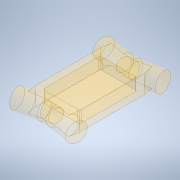
# Autodesk Inventor part: soft_body_v2_simplified
Saved by Autodesk Inventor 2020.2 (Build 242310000, 310)
## iProperties
Created: 2020-07-17
Part Number: soft_body_v2_simplified
Material: Generic
Document SubType Name: Modeling
Designer: boxi
Density: 1 g/cm^3
Appearance: Default
Mass: 1916.47 g
Surface Area: 2811.02 cm^2
Volume: 1916.47 cm^3
Author: boxi
Autodesk Inventor part; units mm, degrees
ref_plane "YZ Plane" through (0, 0, 0) normal (1, 0, 0) x (0, 1, 0)
ref_plane "XY Plane" through (0, 0, 0) normal (0, 0, 1) x (1, 0, 0)
sketch "Sketch1" plane through (0, 0, 0) normal (0, 1, 0) x (-1, 0, 0)
  line L0 (142.9941, 155.2137) -> (0, 130) construction
  line L1 (0, -43.5293) -> (0, 245.4256) projected
  line L2 (256.6466, 0) -> (-100.8661, 0) projected
  line L3 (90.4845, 132.2466) -> (91.6133, 125.8454)
  line L4 (91.6133, 125.8454) -> (98.0145, 126.9741)
  line L5 (98.0145, 126.9741) -> (98.1882, 125.9893)
  line L6 (98.1882, 125.9893) -> (105.0818, 127.2048)
  line L7 (105.0818, 127.2048) -> (106.9919, 116.3719)
  line L8 (106.9919, 116.3719) -> (23.2833, 101.6118)
  line L9 (90.4845, 132.2466) -> (87.5301, 131.7257)
  line L10 (85.5605, 131.3784) -> (86.8629, 123.9923)
  line L11 (86.8629, 123.9923) -> (50.425, 117.5673)
  line L12 (50.425, 117.5673) -> (48.4669, 114.1758)
  line L13 (48.4669, 114.1758) -> (21.8941, 109.4903)
  line L14 (87.5301, 131.7257) -> (89.1103, 122.7639)
  line L15 (89.1103, 122.7639) -> (51.7447, 116.1753)
  line L16 (51.7447, 116.1753) -> (48.7447, 112.6001)
  line L17 (48.7447, 112.6001) -> (22.1719, 107.9146)
  line L18 (21.8941, 109.4903) -> (22.1719, 107.9146)
  line L19 (22.1719, 107.9146) -> (23.2833, 101.6118)
  line L20 (69.4433, 142.2447) -> (75, 110.7309)
  line L21 (75, 107.3146) -> (75, 0)
  line L22 (17.7265, 133.1257) -> (85.1859, 145.0206)
  line L23 (17.7265, 133.1257) -> (21.8941, 109.4903)
  line L24 (87.5301, 131.7257) -> (85.5605, 131.3784)
  line L25 (85.1859, 145.0206) -> (87.5301, 131.7257)
  line L26 (23.2833, 101.6118) -> (0, 101.6118) construction
  line L27 (75, 110.7309) -> (75, 107.3146)
  line L28 (17.7265, 133.1257) -> (0, 130)
  line L29 (67, 0) -> (67, 92.5146)
  line L30 (86.8629, 123.9923) -> (49.4402, 117.3937) construction
  line L31 (49.4402, 117.3937) -> (45.7936, 138.0746) construction
  line L32 (49.4402, 117.3937) -> (39.5921, 115.6572) construction
  line L33 (39.5921, 115.6572) -> (35.9455, 136.3382) construction
  line L34 (39.5921, 115.6572) -> (16.9415, 111.6633) construction
  line L35 (16.9415, 111.6633) -> (13.2949, 132.3443) construction
  line L36 (46.1903, 116.8206) -> (42.5437, 137.5016) construction
  line L37 (42.1526, 116.1087) -> (38.506, 136.7896) construction
  line L38 (0, 55) -> (28, 55)
  line L39 (40, 43) -> (40, 0)
  arc A0 (40, 43) -> (28, 55) centre (28, 43) ccw
  line L40 (75, 107.3146) -> (0, 107.3146)
  line L41 (21.8941, 109.4903) -> (0, 109.4903)
  line L42 (0, 102.5146) -> (57, 102.5146)
  line L43 (17.7265, 133.1257) -> (0, 133.1257)
  line L44 (0, 55) -> (-28, 55)
  line L45 (-40, 43) -> (-40, 0)
  arc A1 (-28, 55) -> (-40, 43) centre (-28, 43) ccw
  line L46 (17.7265, 133.1257) -> (13.559, 156.7611) construction
  line L47 (13.559, 156.7611) -> (46.6849, 162.602) construction
  line L48 (13.559, 156.7611) -> (12.1698, 164.6395) construction
  line L49 (12.1698, 164.6395) -> (95.8785, 179.3996) construction
  line L50 (21.7552, 110.2781) -> (24.5126, 110.7643)
  line L51 (24.5126, 110.7643) -> (25.5905, 110.1421)
  arc A2 (67, 92.5146) -> (57, 102.5146) centre (57, 92.5146) ccw
  line L52 (75, 115.3146) -> (0, 115.3146)
  circle A3 centre (42.5, 0) radius 1.25
  line L53 (45, 0) -> (45, 43)
  arc A4 (45, 43) -> (28, 60) centre (28, 43) ccw
  line L54 (28, 60) -> (0, 60)
  line L55 (0, 60) -> (-28, 60)
  arc A5 (-28, 60) -> (-45, 43) centre (-28, 43) ccw
  line L56 (-45, 43) -> (-45, 0)
  circle A6 centre (42.5, 0) radius 2.25
  line L57 (45, 0) -> (40, 0) construction
  circle A7 centre (0, 57.5) radius 1.25
  circle A8 centre (0, 57.5) radius 2.25
  line L58 (105.0818, 127.2048) -> (101.4352, 147.8858)
  line L59 (85.1859, 145.0206) -> (101.4352, 147.8858)
  line L60 (142.9941, 155.2137) -> (173.3904, -17.1725) construction
  line L61 (12.1698, 164.6395) -> (0, 164.6395) construction
  point P0 (73.3677, 119.9881)
  point P1 (73.0899, 121.5638)
  point P2 (0, 0)
  point P3 (55.6253, 107.3146)
  point P4 (22.2777, 107.3146)
  point P5 (26.6933, 125.6494)
  point P6 (15.6506, 125.6494)
  point P7 (74.1918, 115.3146)
  point P8 (103.6018, 148.2678)
  point P9 (149.94, 115.8214)
  point P10 (74.9102, 105.4662)
  point P11 (0, 59.75)
  point P12 (0, 55.25)
  point P13 (40.25, 0)
  point P14 (44.75, 0)
  dimension "d340" = 10
  dimension "d353" = 1
  dimension "d440" = 10
  dimension "d443" = 10
  dimension "d446" = 4.942
  dimension "d0" = 10
  dimension "d1" = 1
  dimension "d3" = 50
  dimension "d4" = 3
  dimension "d5" = 37
  dimension "d6" = 2
  dimension "d7" = 1.6
  dimension "d9" = 1.6
  dimension "d10" = 42
  dimension "d11" = 6.5
  dimension "d12" = 7
  dimension "d13" = 27
  dimension "d14" = 3
  dimension "d15" = 42
  dimension "d16" = 6.4
  dimension "d17" = 260
  dimension "d24" = 64
  dimension "d27" = 35.4531
  dimension "d63" = 8
  dimension "d67" = 38
  dimension "d68" = 10
  dimension "d69" = 23
  dimension "d77" = 4.1
  dimension "d78" = 3.3
  dimension "d122" = 12
  dimension "d128" = 110
  dimension "d129" = 80
  dimension "d144" = 48
  dimension "d161" = 4.8
  dimension "d190" = 214.6292
  dimension "d193" = 9.4
  dimension "d224" = 45.2
  dimension "d225" = 29.5
  dimension "d226" = 1.6
  dimension "d227" = 40
  dimension "d324" = 40
  dimension "d325" = 0.8
  dimension "d326" = 2.8
  dimension "d456" = 10
  dimension "d468" = 11
  dimension "d469" = 24.3396
  dimension "d513" = 32.4855
  dimension "d514" = 8
  dimension "d520" = 230.6292
  dimension "d538" = 150
  dimension "d539" = 4.5
  dimension "d543" = 0.6
  dimension "d545" = 2.5
  dimension "d546" = 5
  dimension "d548" = 4.5
  dimension "d676" = 2.5
  dimension "d717" = 85
  dimension "d718" = 103
  dimension "d721" = 134
  dimension "d724" = 18
  dimension "d725" = 358.7992
  dimension "d726" = 175.0455
  dimension "d727" = 2.2
  dimension "d728" = 40
  dimension "d729" = 40
  dimension "d730" = 135.0455
  dimension "d731" = 346.7808
  dimension "d732" = 285.9882
  dimension "d733" = 90
  constraints: 120 end point, 14 point on line, 10 point on circle, 9 centre point, 8 horizontal, 6 perpendicular, 4 coincident, 4 horizontal alignment, 4 tangent, 3 equal radius, 3 vertical, 2 collinear, 2 parallel, 1 midpoint, 60 other
  measures "d1" distance between parallel lines of L6 L4
  measures "d3" angle of L12 L11
  measures "d4" distance from line of L13 L11.end
  measures "d5" distance of L10.end L11.end
  measures "d6" distance between parallel lines of L14 L10
  measures "d7" distance between parallel lines of L15 L11
  measures "d9" distance between parallel lines of L17 L13
  measures "d11" distance of L3.end L4.end
  measures "d12" distance of L5.end L6.end
  measures "d14" distance between parallel lines of L3 L14
  measures "d16" distance between parallel lines of L8 L17
  measures "d17" diameter of L28.end L2
  measures "d63" distance between parallel lines of L29 L21
  measures "d67" distance of L10.end L30.end
  measures "d68" distance between parallel lines of L31 L33
  measures "d69" distance of L32.end L34.end
  measures "d77" distance between parallel lines of L36 L37
  measures "d78" distance between parallel lines of L31 L36
  measures "d122" radius of A0
  measures "d128" diameter of L38 L2
  measures "d161" distance between parallel lines of L42 L40
  measures "d190" diameter of L21.start L2
  measures "d193" distance between parallel lines of L8 L15
  measures "d225" distance from line of L23 L11.end
  measures "d226" distance of L16.end L12.end
  measures "d227" angle of L16 L15
  measures "d324" angle of L13 L51
  measures "d325" distance between parallel lines of L13 L50
  measures "d326" distance of L50.start L50.end
  measures "d456" radius of A2
  measures "d468" distance between parallel lines of L8 L6
  measures "d513" distance between parallel lines of L7 L20
  measures "d514" distance from line of L40 L52.start
  measures "d520" diameter of L52.start L2
  measures "d539" distance between parallel lines of L35 L23
  measures "d543" distance from line of L40 L17.end
  measures "d545" diameter of A3
  measures "d546" distance between parallel lines of L39 L53
  measures "d548" diameter of A6
  measures "d676" distance from line of L44 A7.centre
  measures "d717" distance of L58.end L22.start
  measures "d718" distance of L58.end L28.end
  measures "d724" distance of L22.start L28.end
  measures "d725" diameter of L49.end L2
  measures "d727" distance from line of L58 point (103.602, 148.268)
  measures "d728" distance from line of point (103.602, 148.268) L60
  measures "d730" distance of L60.end point (149.94, 115.821)
sketch "Sketch24" plane through (0, 0, 0) normal (0, 1, 0) x (-1, 0, 0)
  line L0 (482.6663, 0) -> (-138.5361, 0) projected
  line L1 (0, -519.9214) -> (0, 362.0665) projected
  line L2 (75, 0) -> (144.4593, -393.9231)
  line L3 (0, 164.6395) -> (393.9231, 234.0988)
  point P0 (0, 0)
  dimension "d736" = 80
  dimension "d737" = 80
  dimension "d740" = 400
  dimension "d741" = 400
  constraints: 4 end point
  measures "d736" angle of L0 L2
  measures "d737" angle of L1 L3
  measures "d740" distance of L2.start L2.end
  measures "d741" distance of L3.start L3.end
sketch "Sketch_3_division_plane" plane through (0, 0, 0) normal (0, 1, 0) x (-1, 0, 0)
  line L0 (17.7265, 133.1257) -> (0, 133.1257) projected
  line L1 (17.7265, 133.1257) -> (172.7798, 160.4657)
  point P0 (0, 0)
  dimension "d207" = 10
  constraints: 2 end point
  measures "d207" angle of L1 L0
ref_plane "Work Plane5" through (-142.9941, 0, 155.2137) normal (0.1736482, 0, 0.9848078) x (0.9848078, 0, -0.1736482)
ref_plane "Work Plane4" through (-17.7265, 0, 133.1257) normal (-0.9848078, 0, 0.1736482) x (0, -1, 0)
ref_plane "Work Plane7" through (-17.7265, 0, 133.1257) normal (0, 0, 1) x (1, 0, 0)
sketch "Sketch2" plane through (-17.7265, 0, 133.1257) normal (-0.9848078, 0, 0.1736482) x (0, -1, 0)
  circle A0 centre (0, 0) radius 32
  circle A1 centre (0, 0) radius 24
  line L0 (-25.6, -10.6039) -> (-25.6, 10.6039)
  line L1 (-25.6, 10.6039) -> (-10.6039, 25.6)
  line L2 (-10.6039, 25.6) -> (10.6039, 25.6)
  line L3 (10.6039, 25.6) -> (25.6, 10.6039)
  line L4 (25.6, 10.6039) -> (25.6, -10.6039)
  line L5 (25.6, -10.6039) -> (10.6039, -25.6)
  line L6 (10.6039, -25.6) -> (-10.6039, -25.6)
  line L7 (-10.6039, -25.6) -> (-25.6, -10.6039)
  point P0 (0, -128.025)
  point P1 (0, 0)
  point P2 (0, 0)
  point P3 (0, 0)
  point P4 (0, -24)
  point P5 (0, -24)
  point P6 (0, -24)
  point P7 (0, -25.6)
  point P8 (0, -25.6)
  point P9 (0, -25.6)
  point P10 (0, -32)
  point P11 (0, -32)
  point P12 (0, -32)
  constraints: 16 end point, 3 coincident, 2 vertical alignment, 1 midpoint, 1 vertical, 21 other
sketch "Sketch3" plane through (0, 0, 0) normal (1, 0, 0) x (0, 1, 0)
  circle A0 centre (0, 133.1257) radius 22.6
  circle A1 centre (0, 133.1257) radius 32
  circle A2 centre (0, 133.1257) radius 28
  dimension "d162" = 64
  dimension "d163" = 45.2
  dimension "d460" = 4
  constraints: 3 centre point, 3 coincident
  measures "d162" diameter of A1
  measures "d163" diameter of A0
  measures "d460" radial gap between concentric circles of A1 A2
sketch "Sketch4" plane through (-142.9941, 0, 155.2137) normal (0.1736482, 0, 0.9848078) x (0.9848078, 0, -0.1736482)
  line L0 (102, 0) -> (106.1, 0) construction
  line L1 (107.55, -16) -> (100.55, -16)
  line L2 (100.55, -16) -> (100.55, 16)
  line L3 (100.55, 16) -> (107.55, 16)
  line L4 (107.55, 16) -> (107.55, -16)
  line L5 (107.55, -16) -> (100.55, 16) construction
  line L6 (100.55, -16) -> (107.55, 16) construction
  circle A0 centre (92.642, 27.3) radius 1.55
  line L7 (0, 0) -> (145.2, 0) construction
  circle A1 centre (92.642, 27.3) radius 1.25
  circle A2 centre (92.642, 27.3) radius 2.5
  line L8 (106.55, 16) -> (106.55, -16)
  line L9 (101.55, 16) -> (101.55, -16)
  line L10 (106.55, 16) -> (101.55, 16)
  line L11 (106.55, 15.3372) -> (106.55, -15.3372)
  line L12 (78.7206, 1.5) -> (77.6794, 1.5)
  line L13 (74.7, 4) -> (74.7, 5)
  line L14 (77.6794, 7.5) -> (78.7206, 7.5)
  line L15 (81.7, 5) -> (81.7, 4)
  line L16 (78.7206, 7.5) -> (81.7, 5)
  line L17 (81.7, 4) -> (78.7206, 1.5)
  line L18 (77.6794, 7.5) -> (74.7, 5)
  line L19 (77.6794, 1.5) -> (74.7, 4)
  line L20 (67.6794, 7.5) -> (64.7, 5)
  line L21 (67.6794, 7.5) -> (68.7206, 7.5)
  line L22 (68.7206, 7.5) -> (71.7, 5)
  line L23 (64.7, 4) -> (64.7, 5)
  line L24 (71.7, 5) -> (71.7, 4)
  line L25 (67.6794, 1.5) -> (64.7, 4)
  line L26 (71.7, 4) -> (68.7206, 1.5)
  line L27 (68.7206, 1.5) -> (67.6794, 1.5)
  line L28 (107.442, -7.8495) -> (106.442, -7.8495)
  line L29 (103.642, -5.5) -> (103.642, -4.5)
  line L30 (106.442, -2.1505) -> (107.442, -2.1505)
  line L31 (110.242, -4.5) -> (110.242, -5.5)
  line L32 (110.242, -5.5) -> (107.442, -7.8495)
  line L33 (110.242, -4.5) -> (107.442, -2.1505)
  line L34 (106.442, -7.8495) -> (103.642, -5.5)
  line L35 (106.442, -2.1505) -> (103.642, -4.5)
  line L36 (110.242, -5) -> (103.642, -5) construction
  line L37 (106.942, -7.8495) -> (106.942, -2.1505) construction
  line L38 (106.442, 2.1505) -> (103.642, 4.5)
  line L39 (103.642, 4.5) -> (103.642, 5.5)
  line L40 (106.442, 7.8495) -> (103.642, 5.5)
  line L41 (106.942, 2.1505) -> (106.942, 7.8495) construction
  line L42 (107.442, 2.1505) -> (106.442, 2.1505)
  line L43 (106.442, 7.8495) -> (107.442, 7.8495)
  line L44 (110.242, 5) -> (103.642, 5) construction
  line L45 (110.242, 4.5) -> (107.442, 2.1505)
  line L46 (110.242, 5.5) -> (110.242, 4.5)
  line L47 (110.242, 5.5) -> (107.442, 7.8495)
  line L48 (118.442, -7.8495) -> (115.642, -5.5)
  line L49 (115.642, -5.5) -> (115.642, -4.5)
  line L50 (118.442, -2.1505) -> (115.642, -4.5)
  line L51 (118.942, -7.8495) -> (118.942, -2.1505) construction
  line L52 (119.442, -7.8495) -> (118.442, -7.8495)
  line L53 (118.442, -2.1505) -> (119.442, -2.1505)
  line L54 (122.242, -5) -> (115.642, -5) construction
  line L55 (122.242, -5.5) -> (119.442, -7.8495)
  line L56 (122.242, -4.5) -> (122.242, -5.5)
  line L57 (122.242, -4.5) -> (119.442, -2.1505)
  line L58 (118.442, 2.1505) -> (115.642, 4.5)
  line L59 (115.642, 4.5) -> (115.642, 5.5)
  line L60 (118.442, 7.8495) -> (115.642, 5.5)
  line L61 (118.942, 2.1505) -> (118.942, 7.8495) construction
  line L62 (119.442, 2.1505) -> (118.442, 2.1505)
  line L63 (118.442, 7.8495) -> (119.442, 7.8495)
  line L64 (122.242, 5) -> (115.642, 5) construction
  line L65 (122.242, 4.5) -> (119.442, 2.1505)
  line L66 (122.242, 5.5) -> (122.242, 4.5)
  line L67 (122.242, 5.5) -> (119.442, 7.8495)
  line L68 (107.55, 13) -> (100.55, 13)
  line L69 (107.55, -13) -> (100.55, -13)
  line L70 (81.7, 4.5) -> (74.7, 4.5) construction
  line L71 (78.7206, -1.5) -> (77.6794, -1.5)
  line L72 (74.7, -4) -> (74.7, -5)
  line L73 (77.6794, -7.5) -> (78.7206, -7.5)
  line L74 (81.7, -5) -> (81.7, -4)
  line L75 (78.7206, -7.5) -> (81.7, -5)
  line L76 (81.7, -4) -> (78.7206, -1.5)
  line L77 (77.6794, -7.5) -> (74.7, -5)
  line L78 (77.6794, -1.5) -> (74.7, -4)
  line L79 (67.6794, -7.5) -> (64.7, -5)
  line L80 (67.6794, -7.5) -> (68.7206, -7.5)
  line L81 (68.7206, -7.5) -> (71.7, -5)
  line L82 (64.7, -4) -> (64.7, -5)
  line L83 (71.7, -5) -> (71.7, -4)
  line L84 (67.6794, -1.5) -> (64.7, -4)
  line L85 (71.7, -4) -> (68.7206, -1.5)
  line L86 (68.7206, -1.5) -> (67.6794, -1.5)
  line L87 (81.7, -4.5) -> (74.7, -4.5) construction
  line L88 (91.7, -4) -> (88.7206, -1.5)
  line L89 (88.7206, 7.5) -> (91.7, 5)
  line L90 (88.7206, -1.5) -> (87.6794, -1.5)
  line L91 (87.6794, -1.5) -> (84.7, -4)
  line L92 (84.7, -4) -> (84.7, -5)
  line L93 (91.7, -4.5) -> (84.7, -4.5) construction
  line L94 (87.6794, -7.5) -> (84.7, -5)
  line L95 (91.7, -5) -> (91.7, -4)
  line L96 (87.6794, -7.5) -> (88.7206, -7.5)
  line L97 (88.7206, -7.5) -> (91.7, -5)
  line L98 (88.7206, 1.5) -> (87.6794, 1.5)
  line L99 (84.7, 4) -> (84.7, 5)
  line L100 (87.6794, 7.5) -> (88.7206, 7.5)
  line L101 (91.7, 5) -> (91.7, 4)
  line L102 (91.7, 4) -> (88.7206, 1.5)
  line L103 (91.7, 4.5) -> (84.7, 4.5) construction
  line L104 (87.6794, 1.5) -> (84.7, 4)
  line L105 (87.6794, 7.5) -> (84.7, 5)
  line L106 (107.55, -16) -> (111.55, -16)
  line L107 (111.55, -16) -> (111.55, 16)
  line L108 (111.55, 16) -> (107.55, 16)
  line L109 (111.55, -5) -> (121.55, -5)
  line L110 (121.55, -5) -> (121.55, 5)
  line L111 (121.55, 5) -> (111.55, 5)
  line L112 (92.642, 27.3) -> (52.642, 27.3)
  circle A3 centre (52.642, 27.3) radius 1.25
  circle A4 centre (52.642, 27.3) radius 1.55
  circle A5 centre (52.642, 27.3) radius 2.5
  point P0 (167.7743, 0)
  point P1 (102, 0)
  point P2 (106.1, 0)
  point P3 (104.05, 0)
  point P4 (96.642, 0)
  point P5 (104.05, 16)
  point P6 (60.7, 0)
  point P7 (81.7, 1.5)
  point P8 (74.7, 7.5)
  point P9 (74.7, 1.5)
  point P10 (81.7, 7.5)
  point P11 (71.7, 7.5)
  point P12 (64.7, 7.5)
  point P13 (64.7, 1.5)
  point P14 (71.7, 1.5)
  point P15 (127.2, 0)
  point P16 (127.2, 0)
  point P17 (127.2, 0)
  point P18 (110.242, -7.8495)
  point P19 (103.642, -2.1505)
  point P20 (103.642, -7.8495)
  point P21 (110.242, -2.1505)
  point P22 (103.642, 2.1505)
  point P23 (103.642, 7.8495)
  point P24 (110.242, 2.1505)
  point P25 (110.242, 7.8495)
  point P26 (115.642, -7.8495)
  point P27 (115.642, -2.1505)
  point P28 (122.242, -7.8495)
  point P29 (122.242, -2.1505)
  point P30 (115.642, 2.1505)
  point P31 (115.642, 7.8495)
  point P32 (122.242, 2.1505)
  point P33 (122.242, 7.8495)
  point P34 (81.7, -1.5)
  point P35 (74.7, -7.5)
  point P36 (74.7, -1.5)
  point P37 (81.7, -7.5)
  point P38 (71.7, -7.5)
  point P39 (64.7, -7.5)
  point P40 (64.7, -1.5)
  point P41 (71.7, -1.5)
  point P42 (84.7, -1.5)
  point P43 (91.7, -1.5)
  point P44 (84.7, -7.5)
  point P45 (91.7, -7.5)
  point P46 (91.7, 1.5)
  point P47 (84.7, 7.5)
  point P48 (84.7, 1.5)
  point P49 (91.7, 7.5)
  dimension "d443" = 10
  dimension "d80" = 7
  dimension "d81" = 32
  dimension "d143" = 54.6
  dimension "d146" = 4
  dimension "d147" = 2.5
  dimension "d148" = 3.1
  dimension "d149" = 5
  dimension "d311" = 5
  dimension "d328" = 7
  dimension "d329" = 6
  dimension "d340" = 10
  dimension "d345" = 4
  dimension "d352" = 2.5
  dimension "d353" = 1
  dimension "d355" = 40
  dimension "d356" = 3
  dimension "d387" = 1
  dimension "d388" = 1
  dimension "d393" = 10
  dimension "d396" = 12
  dimension "d399" = 4.301
  dimension "d400" = 5.4
  dimension "d401" = 40
  dimension "d405" = 7
  dimension "d425" = 3
  dimension "d437" = 3
  dimension "d440" = 10
  dimension "d445" = 3
  dimension "d446" = 4.942
  dimension "d449" = 10
  dimension "d451" = 10
  dimension "d452" = 10
  dimension "d453" = 5.65
  dimension "d464" = 40
  dimension "d542" = 2.8
  constraints: 224 end point, 92 point on line, 74 horizontal alignment, 42 parallel, 26 vertical alignment, 16 collinear, 11 midpoint, 9 perpendicular, 8 equal length, 8 horizontal, 6 centre point, 6 coincident, 3 equal radius, 1 vertical, 33 other
  measures "d80" distance of L1.start L1.end
  measures "d81" distance of L1.end L2.end
  measures "d146" horizontal distance of point (96.642, 0) A0.centre
  measures "d147" diameter of A1
  measures "d148" diameter of A0
  measures "d149" diameter of A2
  measures "d311" distance between parallel lines of L9 L8
  measures "d328" distance of point (81.7, 1.5) point (74.7, 1.5)
  measures "d329" distance of point (74.7, 1.5) point (74.7, 7.5)
  measures "d340" distance of L14.start L20.start
  measures "d345" distance from line of point (60.7, 0) L23
  measures "d352" distance from line of L15.end L12
  measures "d353" distance of L15.start L15.end
  measures "d355" angle of L12 L17
  measures "d356" distance between parallel lines of L24 L13
  measures "d387" distance of L31.start L31.end
  measures "d388" distance of L28.start L28.end
  measures "d393" distance of L28.end L38.start
  measures "d396" distance of L28.end L48.start
  measures "d399" distance between parallel lines of L42 L30
  measures "d400" distance between parallel lines of L31 L49
  measures "d401" angle of L28 L32
  measures "d405" distance from line of point (96.642, 0) L39
  measures "d425" distance between parallel lines of L1 L69
  measures "d437" distance between parallel lines of L71 L12
  measures "d440" distance of L74.end L88.start
  measures "d445" distance between parallel lines of L15 L99
  measures "d446" horizontal distance of L103.start point (96.642, 0)
  measures "d449" distance between parallel lines of L9 L107
  measures "d451" distance of L109.end L110.end
  measures "d452" distance of L110.end L111.end
  measures "d453" distance from line of point (127.2, 0) L110
  measures "d464" distance of L112.start L112.end
  measures "d542" distance from line of L31 L28.start
sketch "Sketch6" plane through (-17.7265, 0, 133.1257) normal (0, 0, 1) x (1, 0, 0)
  circle A0 centre (17.7265, 27.3) radius 1.25
  circle A1 centre (17.7265, 27.3) radius 1.55
  circle A2 centre (17.7265, 27.3) radius 2.5
  line L0 (17.7265, -44.8) -> (17.7265, 44.8) construction
  point P0 (-34.0329, 27.3)
  dimension "d211" = 5
  dimension "d212" = 3.1
  dimension "d213" = 2.5
  dimension "d215" = 0
  constraints: 3 centre point, 2 coincident, 1 horizontal alignment
  measures "d211" diameter of A2
  measures "d212" diameter of A1
  measures "d213" diameter of A0
  measures "d215" distance from line of A0.centre L0
sketch "Sketch11" plane through (0, 0, 0) normal (0, 0, 1) x (1, 0, 0)
  line L0 (-200.7674, 0) -> (91.5529, 0) construction
  line L1 (0, -44.8) -> (0, 44.8) construction
  line L2 (5, 15) -> (-5, 15)
  line L3 (-7, 12.6165) -> (-7, 12.3835)
  line L4 (-5, 10) -> (5, 10)
  line L5 (7, 12.3835) -> (7, 12.6165)
  line L6 (5, 15) -> (7, 12.6165)
  line L7 (-5, 15) -> (-7, 12.6165)
  line L8 (7, 12.3835) -> (5, 10)
  line L9 (-7, 12.3835) -> (-5, 10)
  line L10 (0, 15) -> (0, 10) construction
  line L11 (7, 12.5) -> (-7, 12.5) construction
  line L12 (5, -15) -> (-5, -15)
  line L13 (-7, -12.6165) -> (-7, -12.3835)
  line L14 (-5, -10) -> (5, -10)
  line L15 (7, -12.3835) -> (7, -12.6165)
  line L16 (5, -15) -> (7, -12.6165)
  line L17 (-5, -15) -> (-7, -12.6165)
  line L18 (7, -12.3835) -> (5, -10)
  line L19 (-7, -12.3835) -> (-5, -10)
  line L20 (0, -15) -> (0, -10) construction
  line L21 (7, -12.5) -> (-7, -12.5) construction
  line L22 (-7, -0.1165) -> (-5, -2.5) construction
  line L23 (-5, -2.5) -> (5, -2.5) construction
  line L24 (7, -0.1165) -> (5, -2.5) construction
  line L25 (7, 0) -> (-7, 0) construction
  line L26 (-7, 0.1165) -> (-7, -0.1165) construction
  line L27 (7, -0.1165) -> (7, 0.1165) construction
  line L28 (0, 2.5) -> (0, -2.5) construction
  line L29 (-5, 2.5) -> (-7, 0.1165) construction
  line L30 (5, 2.5) -> (7, 0.1165) construction
  line L31 (5, 2.5) -> (-5, 2.5) construction
  line L32 (5.6995, -4) -> (8.5, -0.6624)
  line L33 (8.5, -0.6624) -> (8.5, 0.6624)
  line L34 (8.5, 0.6624) -> (5.6995, 4)
  line L35 (5.6995, 4) -> (-5.6995, 4)
  line L36 (-5.6995, 4) -> (-8.5, 0.6624)
  line L37 (-8.5, 0.6624) -> (-8.5, -0.6624)
  line L38 (-8.5, -0.6624) -> (-5.6995, -4)
  line L39 (-5.6995, -4) -> (5.6995, -4)
  point P0 (0, 0)
  point P1 (7, 15)
  point P2 (-7, 10)
  point P3 (-7, 15)
  point P4 (7, 10)
  point P5 (7, -15)
  point P6 (-7, -10)
  point P7 (-7, -15)
  point P8 (7, -10)
  point P9 (-7, -2.5)
  point P10 (7, -2.5)
  point P11 (-7, 2.5)
  point P12 (7, 2.5)
  dimension "d470" = 5
  dimension "d471" = 14
  dimension "d480" = 40
  dimension "d481" = 2
  dimension "d482" = 20
  dimension "d491" = 12.5
  dimension "d496" = 7.5
  dimension "d524" = 8
  dimension "d525" = 6
  constraints: 76 end point, 26 point on line, 16 symmetric about line, 4 midpoint, 3 equal length, 2 parallel, 1 horizontal, 1 perpendicular, 1 vertical, 38 other
  measures "d470" distance of point (7, 10) point (7, 15)
  measures "d471" distance of point (7, 15) point (-7, 15)
  measures "d480" angle of L5 L6
  measures "d481" distance of point (7, 15) L2.start
  measures "d482" diameter of L4 L0
  measures "d491" distance of L3.end L22.start
  measures "d496" distance between parallel lines of L31 L4
  measures "d524" distance between parallel lines of L35 L39
  measures "d525" distance between parallel lines of L39 L14
ref_plane "Work Plane11" through (-17.7265, 0, 133.1257) normal (0.9848078, 0, -0.1736482) x (-0.1736482, 0, -0.9848078)
revolve "Revolution4" add sketch "Sketch1" angle 360 about axis through (-142.9941, 0, 155.2137) along (0.9848078, 0, -0.1736482) contours L42 L8 L19 | L19 L40 L8 L42 | L19 L17 L16 L52 L20 L8 L40 | L23 L50 L51 L13 | L13 L12 L52 L16 L17 L18 | L52 L12 L13 L51 L50 L23 | L23 L22 L20 L11 L12 L52 | L20 L15 L14 L9 L3 L4 L5 L6 L7 L8 | L12 L11 L20 L15 L16 L52 | L16 L15 L20 L52 | L22 L25 L24 L10 L11 L20 | L6 L5 L4 L3 L9 L25 L59 L58 | L20 L11 L10 L24 L14 L15
extrude "Extrusion4" add sketch "Sketch1" along normal mid plane 64 contours L54 A4 L53 L2 A6 L39 A0 L38 L1 A8 | L1 L42 L19 L8 A2 L29 L2 L53 A4 L54 | L1 L40 L19 L42 | A8 L1 A7 | L1 L41 L18 L19 L40 | L42 L8 L19 | L19 L40 L8 L42 | A7 L1 | L1 L52 L23 L41 | L19 L17 L16 L52 L20 L8 L40 | L8 L40 L21 L2 L29 A2 L42 | L38 A0 L39 L2 L1 | L1 L28 L23 L52 | L23 L50 L51 L13 | L13 L12 L52 L16 L17 L18 | L8 L27 L40 | L1 L43 L28 | L52 L12 L13 L51 L50 L23 | L23 L22 L20 L11 L12 L52 | L12 L11 L20 L15 L16 L52 | L16 L15 L20 L52 picked at (1.3138, 56.1202) picked at (0.4185, 57.7493)
extrude "Extrusion19" add sketch "Sketch3" against normal through all contours A0 | A1 | A2
extrude "Extrusion6-body begin" add sketch "Sketch1" along normal mid plane 64 contours L54 A4 L53 L2 A6 L39 A0 L38 L1 A8 | L1 L42 L19 L8 A2 L29 L2 L53 A4 L54 | L1 L40 L19 L42 | A8 L1 A7 | L42 L8 L19 | L19 L40 L8 L42 | A7 L1 | L8 L40 L21 L2 L29 A2 L42 | L38 A0 L39 L2 L1 | L2 A3 A6 | L2 A3 picked at (1.3138, 56.1202) picked at (0.4185, 57.7493) picked at (40.6051, 0.1795) picked at (42.8596, 0.4699)
extrude "Extrusion7_hollow mid body" cut sketch "Sketch1" along normal mid plane 48 contours L54 A4 L53 L2 A6 L39 A0 L38 L1 A8 | L1 L42 L19 L8 A2 L29 L2 L53 A4 L54 | A8 L1 A7 | L42 L8 L19 | A7 L1 | L38 A0 L39 L2 L1 | L2 A3 A6 | L2 A3 picked at (1.3138, 56.1202) picked at (0.4185, 57.7493) picked at (40.6051, 0.1795) picked at (42.8596, 0.4699)
extrude "Extrusion48_hollow_front_body" cut sketch "Sketch3" against normal up to surface contours A0 surface through (-17.7265, 0, 133.1257) normal (0.9848078, 0, -0.1736482)
mirror "Mirror14" about plane through (0, 0, 0) normal (1, 0, 0)
extrude "Extrusion50" [suppressed]
thicken "Thicken81_simulation_compensation" operation add thickness 4 both sides no extend neighbours yes toward (-1, 0, 0) faces at (67, -8, 30.8382) (66.972, -8, 93.2619) (-38, 8, 102.5146) (38, 8, 102.5146) (-66.972, -8, 93.2619) (-67, -8, 30.8382) (-22.3333, -24, 65.0097) (22.3333, -24, 65.0097) (-22.3333, 24, 65.0097) (22.3333, 24, 65.0097)
mirror "Mirror15" about plane through (0, 0, 0) normal (0, 0, 1)
equation "\"d15\" = d10"
equation "\"motor_angle\" = 10deg"
equation "\"wall_thickness\" = 8"
equation "\"shrink_compensation\" = 0.38"
equation "\"thicken_skin\" = 0.4"
equation "\"thicken_skin_screw\" = 1.6"
equation "\"d27_Copy\" = 35.45308"
body "Solid1"
body "Srf8"
body "Srf9"
body "Srf12"
body "Srf13"
